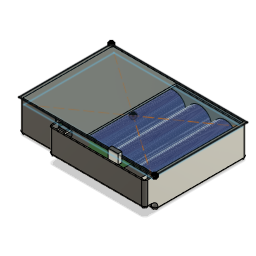
Luna Laser Box v3 (Autodesk Fusion 360 design; units mm, degrees)
Autodesk Fusion 360 part; units mm, degrees
sketch "Sketch9" plane through (0, 0, 0) normal (0, 1, 0) x (1, 0, 0)
  line L0 (53, 36) -> (-53, 36)
  line L1 (-53, 36) -> (-53, -36)
  line L2 (-53, -36) -> (53, -36)
  line L3 (53, -36) -> (53, 36)
  line L4 (53, 36) -> (-53, -36) construction
  line L5 (-53, 36) -> (53, -36) construction
  dimension "d23" = 106
  dimension "d24" = 72
  constraint horizontal L0
  constraint perpendicular L0 L1
  constraint parallel L0 L2
  constraint parallel L1 L3
  constraint coincident L4 origin
  constraint coincident L5 origin
  measures "d23" distance of L1.end L2.end
  measures "d24" distance of L0.end L1.end
extrude "Extrude6" add sketch "Sketch9" along normal blind 25 makes body 1
sketch "Sketch10" plane through (0, 25, 0) normal (0, 1, 0) x (-1, 0, 0)
  line L0 (-53, 36) -> (-53, -36)
  line L1 (-53, -36) -> (53, -36)
  line L2 (53, -36) -> (53, 36)
  line L3 (53, 36) -> (-53, 36)
  line L4 (-51, 34) -> (51, 34)
  line L5 (51, 34) -> (51, -34)
  line L6 (51, -34) -> (-51, -34)
  line L7 (-51, -34) -> (-51, 34)
  line L8 (-51, 34) -> (51, -34) construction
  line L9 (51, 34) -> (-51, -34) construction
  dimension "d27" = 102
  dimension "d28" = 68
  constraint horizontal L4
  constraint perpendicular L4 L5
  constraint parallel L4 L6
  constraint parallel L5 L7
  constraint coincident L8 origin
  constraint coincident L9 origin
  measures "d27" distance of L5.end L6.end
  measures "d28" distance of L4.end L5.end
extrude "Extrude7" cut sketch "Sketch10" against normal blind 23 contours L4 L5 L6 L7 bodies 1
sketch "Sketch13" plane through (0, 25, 0) normal (0, 1, 0) x (-1, 0, 0)
  line L0 (51, 34) -> (51, -34)
  line L1 (51, -34) -> (-51, -34)
  line L2 (-51, -34) -> (-51, 34)
  line L3 (-51, 34) -> (51, 34)
  line L4 (-53, 36) -> (-53, -36)
  line L5 (-53, -36) -> (53, -36)
  line L6 (53, -36) -> (53, 36)
  line L7 (53, 36) -> (-53, 36)
  line L8 (53, -36) -> (-53, -36)
  line L9 (-53, -36) -> (-53, 36)
  line L10 (-53, 36) -> (53, 36)
  line L11 (53, 36) -> (53, -36)
  constraint horizontal L8
  constraint vertical L9
  constraint horizontal L10
  constraint vertical L11
  constraint coincident L4.start L7.end
  constraint coincident L5.end L6.start
ref_plane "WorkPlane3" through (0, 21, 0) normal (0, 1, 0) x (-1, 0, 0)
sketch "Sketch15" plane through (0, 21, 0) normal (0, 1, 0) x (1, 0, 0)
  line L0 (50, -35) -> (-50, -35)
  line L1 (-50, -35) -> (-50, 35)
  line L2 (-50, 35) -> (50, 35)
  line L3 (50, 35) -> (50, -35)
  line L4 (50, -35) -> (-50, 35) construction
  line L5 (-50, -35) -> (50, 35) construction
  constraint horizontal L0
  constraint perpendicular L0 L1
  constraint parallel L0 L2
  constraint parallel L1 L3
  constraint coincident L4 origin
  constraint coincident L5 origin
sketch "Sketch16" plane through (-53, 0, 0) normal (-1, 0, 0) x (0, 0, 1)
  line L0 (-36, 0) -> (36, 0)
  line L1 (36, 0) -> (36, 25)
  line L2 (36, 25) -> (-36, 25)
  line L3 (-36, 25) -> (-36, 0)
  circle A0 centre (75, 15) radius 9.2
  dimension "d34" = 18.4
  measures "d34" diameter of A0
extrude "Extrude8" add sketch "Sketch16" against normal blind 64 separate body contours A0 makes body 2
fillet "Fillet4" radius 1 1 edges at (11, 18.3269, 66.4226) on bodies 2
move_body "Move1" bodies 2 to x (0, -0.007964, 0.999968) y (-0.251118, 0.967926, 0.007709) z (-0.967956, -0.25111, -0.002) at (113.7895, 16.8471, 19.05)
copy_body "CopyPasteBodies1" bodies 2 makes body 3
move_body "Move2" bodies 3 to x (1, 0, 0) y (0, 1, 0) z (0, 0, 1) at (-20, 0, 0)
copy_body "CopyPasteBodies2" bodies 3 2 makes body 4 makes body 5
move_body "Move3" bodies 4 5 to x (1, 0, 0) y (0, 1, 0) z (0, 0, 1) at (-40, 0, 0)
copy_body "CopyPasteBodies3" bodies 4 makes body 6
move_body "Move4" bodies 6 to x (1, 0, 0) y (0, 1, 0) z (0, 0, 1) at (-20, 0, 0)
move_body "Move5" bodies 2 3 4 5 6 to x (1, 0, 0) y (0, 1, 0) z (0, 0, 1) at (2.5, 0, 0)
move_body "Move6" bodies 2 3 4 5 6 to x (1, 0, 0) y (0, 1, 0) z (0, 0, 1) at (0, 0, 2)
sketch "Sketch17" plane through (0, 0, 36) normal (0, 0, 1) x (1, 0, 0)
  line L0 (-53, 0) -> (53, 0)
  line L1 (53, 0) -> (53, 25)
  line L2 (53, 25) -> (-53, 25)
  line L3 (-53, 25) -> (-53, 0)
  line L4 (110, 25) -> (181.5, 25)
  line L5 (181.5, 25) -> (181.5, 7)
  line L6 (181.5, 7) -> (110, 7)
  line L7 (110, 7) -> (110, 25)
  dimension "d39" = 71.5
  dimension "d40" = 18
  constraint horizontal L4
  constraint vertical L5
  constraint horizontal L6
  constraint vertical L7
  measures "d39" distance of L4.start L4.end
  measures "d40" distance of L4.start L6.end
extrude "Extrude9" add sketch "Sketch17" against normal blind 1 separate body contours L4 L5 L6 L7 makes body 7
sketch "Sketch18" plane through (0, 0, 36) normal (0, 0, 1) x (1, 0, 0)
  line L0 (110, 7) -> (181.5, 7)
  line L1 (181.5, 7) -> (181.5, 25)
  line L2 (181.5, 25) -> (110, 25)
  line L3 (110, 25) -> (110, 7)
  line L4 (178, 24) -> (164.7, 24)
  line L5 (164.7, 24) -> (164.7, 10.2)
  line L6 (164.7, 10.2) -> (178, 10.2)
  line L7 (178, 10.2) -> (178, 24)
  dimension "d43" = 13.3
  dimension "d44" = 13.8
  constraint horizontal L4
  constraint vertical L5
  constraint horizontal L6
  constraint vertical L7
  measures "d43" distance of L4.start L4.end
  measures "d44" distance of L4.start L6.end
extrude "Extrude10" add sketch "Sketch18" along normal blind 5 contours L4 L5 L6 L7 bodies 7
sketch "Sketch19" plane through (0, 0, 36) normal (0, 0, 1) x (1, 0, 0)
  line L0 (178, 10.2) -> (164.7, 10.2)
  line L1 (164.7, 10.2) -> (164.7, 24)
  line L2 (164.7, 24) -> (178, 24)
  line L3 (178, 24) -> (178, 10.2)
  line L4 (110, 7) -> (181.5, 7)
  line L5 (181.5, 7) -> (181.5, 25)
  line L6 (181.5, 25) -> (110, 25)
  line L7 (110, 25) -> (110, 7)
  line L8 (158.2778, 21.8674) -> (150.4778, 21.8674)
  line L9 (150.4778, 21.8674) -> (150.4778, 29.3674)
  line L10 (150.4778, 29.3674) -> (158.2778, 29.3674)
  line L11 (158.2778, 29.3674) -> (158.2778, 21.8674)
  dimension "d47" = 7.8
  dimension "d48" = 7.5
  constraint horizontal L8
  constraint vertical L9
  constraint horizontal L10
  constraint vertical L11
  measures "d47" distance of L8.start L8.end
  measures "d48" distance of L8.start L10.end
extrude "Extrude11" add sketch "Sketch19" along normal blind 3 contours L6 L9 L10 L11 | L6 L8 L9 L11 bodies 7
sketch "Sketch20" plane through (0, 0, 36) normal (0, 0, 1) x (1, 0, 0)
  line L0 (150.4778, 21.8674) -> (150.4778, 25)
  line L1 (150.4778, 25) -> (110, 25)
  line L2 (110, 25) -> (110, 7)
  line L3 (110, 7) -> (181.5, 7)
  line L4 (181.5, 7) -> (181.5, 25)
  line L5 (181.5, 25) -> (158.2778, 25)
  line L6 (158.2778, 25) -> (158.2778, 21.8674)
  line L7 (158.2778, 21.8674) -> (150.4778, 21.8674)
  line L8 (178, 10.2) -> (164.7, 10.2)
  line L9 (164.7, 10.2) -> (164.7, 24)
  line L10 (164.7, 24) -> (178, 24)
  line L11 (178, 24) -> (178, 10.2)
  line L12 (112, 24) -> (119.3, 24)
  line L13 (119.3, 24) -> (119.3, 20.4)
  line L14 (119.3, 20.4) -> (112, 20.4)
  line L15 (112, 20.4) -> (112, 24)
  dimension "d51" = 7.3
  dimension "d52" = 3.6
  constraint horizontal L12
  constraint vertical L13
  constraint horizontal L14
  constraint vertical L15
  measures "d51" distance of L12.start L12.end
  measures "d52" distance of L12.start L14.end
extrude "Extrude12" add sketch "Sketch20" along normal blind 5 contours L12 L13 L14 L15 bodies 7
sketch "Sketch21" plane through (0, 24, 0) normal (0, 1, 0) x (-1, 0, 0)
  line L0 (-119.3, 36) -> (-112, 36)
  line L1 (-112, 36) -> (-112, 41)
  line L2 (-112, 41) -> (-119.3, 41)
  line L3 (-119.3, 41) -> (-119.3, 36)
  line L4 (-113, 37) -> (-118, 37)
  line L5 (-118, 37) -> (-118, 40)
  line L6 (-118, 40) -> (-113, 40)
  line L7 (-113, 40) -> (-113, 37)
  constraint horizontal L4
  constraint vertical L5
  constraint horizontal L6
  constraint vertical L7
extrude "Extrude13" add sketch "Sketch21" along normal blind 1.5 contours L4 L5 L6 L7 bodies 7
move_body "Move7" bodies 7 to x (1, 0, 0) y (0, 1, 0) z (0, 0, 1) at (-130, 0, 1)
sketch "Sketch22" plane through (0, 25, 0) normal (0, 1, 0) x (-1, 0, 0)
  line L0 (51, -35) -> (-51, -35)
  line L1 (-51, -35) -> (-51, 35)
  line L2 (-51, 35) -> (51, 35)
  line L3 (51, 35) -> (51, -35)
  line L4 (51, -35) -> (-51, 35) construction
  line L5 (-51, -35) -> (51, 35) construction
  line L6 (25, -35) -> (-25, -35)
  line L7 (-25, -35) -> (-25, 35)
  line L8 (-25, 35) -> (25, 35)
  line L9 (25, 35) -> (25, -35)
  line L10 (25, -35) -> (-25, 35) construction
  line L11 (-25, -35) -> (25, 35) construction
  dimension "d57" = 102
  dimension "d58" = 70
  dimension "d61" = 50
  constraint horizontal L0
  constraint perpendicular L0 L1
  constraint parallel L0 L2
  constraint parallel L1 L3
  constraint coincident L4 origin
  constraint coincident L5 origin
  constraint horizontal L6
  constraint perpendicular L6 L7
  constraint parallel L6 L8
  constraint parallel L7 L9
  constraint coincident L10 origin
  constraint coincident L11 origin
  measures "d57" distance of L1.end L2.end
  measures "d58" distance of L0.end L1.end
  measures "d61" distance of L7.end L8.end
extrude "Extrude14" cut sketch "Sketch22" against normal blind 1.5 bodies 1
sketch "Sketch23" plane through (0, 25, 0) normal (0, 1, 0) x (-1, 0, 0)
  line L0 (155, 35) -> (105, 35)
  line L1 (105, 35) -> (105, -35)
  line L2 (105, -35) -> (155, -35)
  line L3 (155, -35) -> (155, 35)
  line L4 (155, 35) -> (105, -35) construction
  line L5 (105, 35) -> (155, -35) construction
  point P0 (130, 0)
  dimension "d62" = 50
  dimension "d63" = 70
  constraint horizontal L0
  constraint perpendicular L0 L1
  constraint parallel L0 L2
  constraint parallel L1 L3
  constraint coincident L4 P0
  constraint coincident L5 P0
  measures "d62" distance of L1.end L2.end
  measures "d63" distance of L0.end L1.end
extrude "Extrude15" add sketch "Sketch23" against normal blind 1.5 separate body makes body 8
move_face "MoveFace1" by (100, 0, 0) 1 faces at (-121.6667, 25, 11.6667) on bodies 8
move_face "MoveFace2" by (60, 0, 0) 1 faces at (-121.6667, 25, 11.6667) on bodies 8
move_body "Move8" bodies 8 to x (1, 0, 0) y (0, 1, 0) z (0, 0, 1) at (50, 0, 0)
move_body "Move9" bodies 8 to x (1, 0, 0) y (0, 1, 0) z (0, 0, 1) at (54, 0, 0)
sketch "Sketch24" plane through (0, 0, 36) normal (0, 0, 1) x (1, 0, 0)
  line L0 (-53, 0) -> (53, 0)
  line L1 (53, 0) -> (53, 25)
  line L2 (53, 25) -> (-53, 25)
  line L3 (-53, 25) -> (-53, 0)
  line L4 (53, 25) -> (-22, 25)
  line L5 (-22, 25) -> (-22, 5)
  line L6 (-22, 5) -> (53, 5)
  line L7 (53, 5) -> (53, 25)
  dimension "d66" = 75
  dimension "d67" = 20
  constraint horizontal L4
  constraint vertical L5
  constraint horizontal L6
  constraint vertical L7
  constraint coincident L1.end L2.start
  measures "d66" distance of L1.end L4.end
  measures "d67" distance of L1.end L6.end
move_body "Move10" bodies 7 to x (1, 0, 0) y (0, 1, 0) z (0, 0, 1) at (100, 0, 0)
extrude "Extrude16" add sketch "Sketch24" along normal blind 8 contours L1 L2 L4 L5 L6 L7 bodies 1
sketch "Sketch25" plane through (0, 25, 0) normal (0, 1, 0) x (-1, 0, 0)
  line L0 (-53, 44) -> (-53, -36)
  line L1 (-53, -36) -> (53, -36)
  line L2 (53, -36) -> (53, 36)
  line L3 (53, 36) -> (22, 36)
  line L4 (22, 36) -> (22, 44)
  line L5 (22, 44) -> (-53, 44)
  line L6 (-51, -35) -> (-51, 35)
  line L7 (-51, 35) -> (51, 35)
  line L8 (51, 35) -> (51, -35)
  line L9 (51, -35) -> (-51, -35)
  line L10 (21, 37) -> (-52, 37)
  line L11 (-52, 37) -> (-52, 43)
  line L12 (-52, 43) -> (21, 43)
  line L13 (21, 43) -> (21, 37)
  constraint horizontal L10
  constraint vertical L11
  constraint horizontal L12
  constraint vertical L13
extrude "Extrude17" cut sketch "Sketch25" against normal blind 19 contours L10 L11 L12 L13 bodies 1
sketch "Sketch26" plane through (0, 0, 37) normal (0, 0, 1) x (1, 0, 0)
  line L0 (52, 25) -> (-21, 25)
  line L1 (-21, 25) -> (-21, 6)
  line L2 (-21, 6) -> (52, 6)
  line L3 (52, 6) -> (52, 25)
  circle A0 centre (6, 9) radius 2
extrude "Extrude18" cut sketch "Sketch26" against normal blind 16 contours A0 bodies 1 5
move_body "Move11" bodies 7 to x (1, 0, 0) y (0, 1, 0) z (0, 0, 1) at (-100, 0, 0)
fillet "Fillet6" radius 2.4 15 edges at (0, 0, 36) (-53, 0, 0) (53, 0, 0) (0, 0, -36) (53, 2.5, 36) (53, 5, 40) (15.5, 5, 44) (53, 15, 44) (-22, 15, 44) (-22, 15, 36) (-53, 12.5, 36) (-53, 12.5, -36) (53, 12.5, -36) (-22, 5, 40) (15.5, 5, 36) on bodies 1
named bodies: "Box", "Circuit charger", "Lid"
